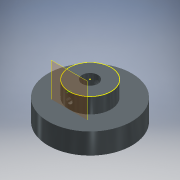
# Autodesk Inventor part: Clamp Knob
Saved by Autodesk Inventor 2020 (Build 240168000, 168)
## iProperties
Created: 2019-11-14
Part Number: Clamp Knob
Material: Iron, Cast
Document SubType Name: Modeling
Designer: Jorge
Density: 7.15 g/cm^3
Appearance: Iron Gray
Author: Jorge
Autodesk Inventor part; units mm, degrees
ref_plane "YZ Plane" through (0, 0, 0) normal (1, 0, 0) x (0, 1, 0)
ref_plane "XZ Plane" through (0, 0, 0) normal (0, 1, 0) x (-1, 0, 0)
ref_plane "XY Plane" through (0, 0, 0) normal (0, 0, 1) x (1, 0, 0)
sketch "Sketch1" plane through (0, 0, 0) normal (1, 0, 0) x (0, 1, 0)
  line L0 (22.225, 4.7625) -> (22.225, 12.7)
  line L1 (22.225, 12.7) -> (12.7, 12.7)
  line L2 (12.7, 12.7) -> (12.7, 25.4)
  line L3 (12.7, 25.4) -> (0, 25.4)
  line L4 (0, 25.4) -> (0, 4.7625)
  line L5 (0, 4.7625) -> (22.225, 4.7625)
  line L6 (-4.445, 0) -> (26.67, 0) projected
  line L7 (0, -5.08) -> (0, 30.48) construction
  point P0 (0, 0)
  dimension "d0" = 25.4
  dimension "d1" = 9.525
  dimension "d2" = 22.225
  dimension "d4" = 12.7
  dimension "d5" = 50.8
  constraints: 12 end point, 5 perpendicular, 1 collinear, 1 vertical
  measures "d0" diameter of L1 L6
  measures "d1" diameter of L5 L6
  measures "d2" distance between parallel lines of L0 L7
  measures "d4" distance between parallel lines of L2 L7
  measures "d5" diameter of L3 L6
revolve "Revolution1" add sketch "Sketch1" angle 360 about axis through (0, -10, 0) along (0, 1, 0)
sketch "Sketch2" plane through (0, 22.225, 0) normal (0, 1, 0) x (1, 0, 0)
  circle A0 centre (0, 0) radius 12.7 projected
  point P0 (0, -12.7)
  constraints: 1 vertical alignment, 1 other
ref_plane "Work Plane1" through (0, 22.225, 12.7) normal (0, 0, 1) x (1, 0, 0)
sketch "Sketch3" plane through (0, 22.225, 12.7) normal (0, 0, 1) x (1, 0, 0)
  line L0 (12.7, 0) -> (-12.7, 0) projected
  point P0 (0, -22.225)
  point P1 (0, -4.7625)
  dimension "d7" = 4.7625
  measures "d7" distance from line of point (0, -4.763) L0
hole "Hole1" at (0, 17.4625, 12.7) direction (0, 0, -1) diameter 3.8608 end through all
body "Solid1"
